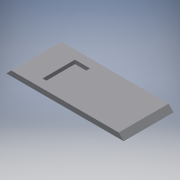
# Autodesk Inventor part: deksel token Nieuw bevestiging
Saved by Autodesk Inventor 2018.3 (Build 223284000, 284)
## iProperties
Created: 2020-11-30
Part Number: deksel token Nieuw bevestiging
Material: Generic
Document SubType Name: Modeling
Designer: Olivi
Density: 1 g/cm^3
Appearance: Default
Author: Olivi
Autodesk Inventor part; units mm, degrees
ref_plane "YZ Plane" through (0, 0, 0) normal (1, 0, 0) x (0, 1, 0)
ref_plane "XZ Plane" through (0, 0, 0) normal (0, 1, 0) x (-1, 0, 0)
ref_plane "XY Plane" through (0, 0, 0) normal (0, 0, 1) x (1, 0, 0)
sketch "Sketch1" plane through (0, 0, 0) normal (0, 0, 1) x (1, 0, 0)
  line L0 (0, 0) -> (43, 0)
  line L1 (43, 0) -> (43, 20)
  line L2 (43, 20) -> (0, 20)
  line L3 (0, 20) -> (0, 0)
  dimension "d0" = 43
  dimension "d1" = 20
  constraints: 8 end point, 2 parallel, 1 horizontal, 1 perpendicular
  measures "d0" distance of L2.end L1.end
  measures "d1" distance of L1.end L0.end
extrude "Extrusion1" add sketch "Sketch1" along normal blind 2
sketch "Sketch2" plane through (0, 0, 0) normal (0, -1, 0) x (1, 0, 0)
  line L0 (43, 0) -> (43, 2) projected
  line L1 (0, 0) -> (0, 2) projected
  line L2 (0, 0) -> (-2, 0)
  line L3 (-2, 0) -> (0, 2)
  line L4 (43, 0) -> (45, 0)
  line L5 (45, 0) -> (43, 2)
  dimension "d4" = 2
  dimension "d5" = 2
  constraints: 8 end point, 2 horizontal
  measures "d4" distance of L1.start L2.end
  measures "d5" distance of L0.start L4.end
extrude "Extrusion2" add sketch "Sketch2" against normal blind 20
sketch "Sketch3" plane through (0, 0, 2) normal (0, 0, 1) x (1, 0, 0)
  line L0 (0, 0) -> (43, 0) projected
  line L1 (43, 0) -> (43, 20) projected
  line L2 (43, 20) -> (0, 20) projected
  line L3 (0, 20) -> (0, 0) projected
  line L4 (9, 3.5) -> (34, 3.5)
  line L5 (34, 3.5) -> (34, 16.5)
  line L6 (34, 16.5) -> (9, 16.5)
  line L7 (9, 16.5) -> (9, 3.5)
  dimension "d8" = 25
  dimension "d9" = 13
  dimension "d10" = 3.5
  dimension "d11" = 3.5
  dimension "d12" = 9
  dimension "d13" = 9
  constraints: 8 end point, 2 parallel, 1 horizontal, 1 perpendicular
  measures "d8" distance of L6.end L5.end
  measures "d9" distance of L5.end L4.end
  measures "d10" distance between parallel lines of L0 L4
  measures "d11" distance between parallel lines of L2 L6
  measures "d12" distance between parallel lines of L1 L5
  measures "d13" distance between parallel lines of L3 L7
extrude "Extrusion3" cut sketch "Sketch3" against normal blind 1.5 contours L7 L6 L5 L4
sketch "Sketch4" plane through (0, 0, 2) normal (0, 0, 1) x (1, 0, 0)
  line L0 (34, 16.5) -> (34, 3.5) projected
  line L1 (34, 3.5) -> (15, 3.5)
  line L2 (15, 3.5) -> (15, 8)
  line L3 (15, 8) -> (34, 8)
  line L4 (34, 8) -> (34, 3.5)
  line L5 (9, 16.5) -> (34, 16.5) projected
  line L6 (34, 16.5) -> (15, 16.5)
  line L7 (15, 16.5) -> (15, 12)
  line L8 (15, 12) -> (34, 12)
  line L9 (34, 12) -> (34, 16.5)
  dimension "d16" = 19
  dimension "d17" = 4.5
  dimension "d18" = 4.5
  constraints: 16 end point, 4 parallel, 2 horizontal, 2 perpendicular
  measures "d16" distance of L2.end L3.end
  measures "d17" distance of L1.end L2.end
  measures "d18" distance of L7.end L6.end
extrude "Extrusion4" add sketch "Sketch4" against normal blind 1.49
chamfer "Chamfer5" distance 4.5 distance2 1.49 1 edges at (24.5, 12, 0.51) measured on face at (24.5, 12.5, 0.51)
chamfer "Chamfer6" distance 4.5 distance2 1.49 1 edges at (24.5, 8, 0.51) measured on face at (24.5, 7.5, 0.51)
body "Solid1"
